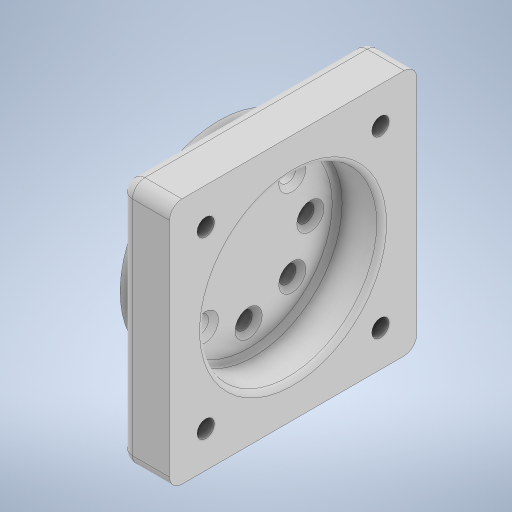
# Autodesk Inventor part: adaptador para Kuka
Saved by Autodesk Inventor 2024 (Build 280153000, 153)
## iProperties
Created: 2026-04-16
Part Number: adaptador para Kuka
Material: Genérico
Document SubType Name: Modeling
Designer: Legion
Density: 1 g/cm^3
Appearance: Valor por defecto
Author: Legion
Autodesk Inventor part; units mm, degrees
ref_plane "YZ Plane" through (0, 0, 0) normal (1, 0, 0) x (0, 1, 0)
ref_plane "XZ Plane" through (0, 0, 0) normal (0, 1, 0) x (-1, 0, 0)
ref_plane "XY Plane" through (0, 0, 0) normal (0, 0, 1) x (1, 0, 0)
sketch "Boceto1" plane through (0, 0, 0) normal (1, 0, 0) x (0, 1, 0)
  circle A0 centre (0, 0) radius 31.7
  circle A1 centre (0, 0) radius 40
  dimension "d0" = 63.4
  dimension "d1" = 80
  constraints: 2 centre point, 2 coincident
  measures "d0" diameter of A0
  measures "d1" diameter of A1
extrude "Extrusión1" add sketch "Boceto1" along normal blind 10 contours A0 | A1
extrude "Extrusión2" cut sketch "Boceto1" along normal blind 5 contours A0
sketch "Boceto2" plane through (10, 0, 0) normal (1, 0, 0) x (0, 0, -1)
  line L0 (0, 0) -> (50, 0)
  line L1 (0, 0) -> (-50, 0)
  line L2 (0, 0) -> (0, -50)
  line L3 (0, 0) -> (0, 50)
  line L4 (50, 50) -> (-50, 50)
  line L5 (-50, 50) -> (-50, -50)
  line L6 (-50, -50) -> (50, -50)
  line L7 (50, -50) -> (50, 50)
  dimension "d6" = 50
  dimension "d7" = 50
  dimension "d8" = 50
  dimension "d9" = 50
  constraints: 16 end point, 3 horizontal, 2 parallel, 2 perpendicular, 1 vertical
  measures "d6" distance of L0.start L0.end
  measures "d7" distance of L0.start L1.end
  measures "d8" distance of L0.start L2.end
  measures "d9" distance of L0.start L3.end
extrude "Extrusión3" add sketch "Boceto2" along normal blind 20
sketch "Boceto3" plane through (30, 0, 0) normal (1, 0, 0) x (0, 0, -1)
  circle A0 centre (0, 0) radius 31.7 projected
  circle A1 centre (0, 0) radius 40 projected
  circle A2 centre (0, 0) radius 31.7 projected
  line L0 (31.7, 0) -> (40, 0)
  circle A3 centre (0, 0) radius 35.85
  constraints: 2 end point, 2 horizontal alignment, 1 centre point, 1 coincident, 1 horizontal, 2 other
extrude "Extrusión4" cut sketch "Boceto3" against normal blind 18 contours A0 | A3
sketch "Boceto4" plane through (12, 0, 0) normal (1, 0, 0) x (0, 0, -1)
  circle A0 centre (0, 0) radius 25
  line L0 (-17.6777, -17.6777) -> (17.6777, 17.6777)
  line L1 (0, 0) -> (25, 0) construction
  line L2 (-17.6777, 17.6777) -> (17.6777, -17.6777)
  point P0 (0, -25)
  point P1 (-25, 0)
  point P2 (0, 25)
  dimension "d14" = 50
  dimension "d15" = 45
  constraints: 6 coincident, 6 end point, 2 midpoint, 1 horizontal, 9 other
  measures "d15" angle of L1 L0
hole "Agujero1" at (12, 17.6777, -17.6777) at (12, 0, -25) at (12, -17.6777, -17.6777) at (12, -25, 0) at (12, -17.6777, 17.6777) at (12, 0, 25) at (12, 17.6777, 17.6777) at (12, 25, 0) direction (-1, 0, 0) diameter 7 end through all countersink diameter 11 countersink angle 90
sketch "Boceto5" plane through (30, 0, 0) normal (1, 0, 0) x (0, 0, -1)
  circle A0 centre (0, 0) radius 50
  line L0 (50, 50) -> (-35.3553, -35.3553)
  line L1 (-35.3553, 35.3553) -> (50, -50)
  point P0 (35.3553, 35.3553)
  point P1 (-35.3553, -35.3553)
  point P2 (35.3553, -35.3553)
  constraints: 4 end point, 4 point on circle, 4 point on line, 3 coincident, 1 centre point
hole "Agujero2" at (30, 35.3553, -35.3553) at (30, 35.3553, 35.3553) at (30, -35.3553, 35.3553) at (30, -35.3553, -35.3553) direction (-1, 0, 0) diameter 7 end through all
sketch "Boceto6" plane through (10, 0, 0) normal (-1, 0, 0) x (0, 0, 1)
  circle A0 centre (-35.3553, -35.3553) radius 3.5
  line L0 (-37.6553, -39.3391) -> (-39.9553, -35.3553)
  line L1 (-39.9553, -35.3553) -> (-37.6553, -31.3716)
  line L2 (-37.6553, -31.3716) -> (-33.0553, -31.3716)
  line L3 (-33.0553, -31.3716) -> (-30.7553, -35.3553)
  line L4 (-30.7553, -35.3553) -> (-33.0553, -39.3391)
  line L5 (-33.0553, -39.3391) -> (-37.6553, -39.3391)
  line L6 (-35.3553, -35.3553) -> (-39.9553, -35.3553)
  circle A1 centre (-35.3553, 35.3553) radius 3.5
  circle A2 centre (35.3553, 35.3553) radius 3.5
  circle A3 centre (35.4038, -35.3068) radius 3.5
  line L7 (-37.6553, 31.3716) -> (-39.9553, 35.3553)
  line L8 (-33.0553, 31.3716) -> (-37.6553, 31.3716)
  line L9 (-30.7553, 35.3553) -> (-33.0553, 31.3716)
  line L10 (-33.0553, 39.3391) -> (-30.7553, 35.3553)
  line L11 (-37.6553, 39.3391) -> (-33.0553, 39.3391)
  line L12 (-39.9553, 35.3553) -> (-37.6553, 39.3391)
  line L13 (33.0553, 31.3716) -> (30.7553, 35.3553)
  line L14 (37.6553, 31.3716) -> (33.0553, 31.3716)
  line L15 (39.9553, 35.3553) -> (37.6553, 31.3716)
  line L16 (37.6553, 39.3391) -> (39.9553, 35.3553)
  line L17 (33.0553, 39.3391) -> (37.6553, 39.3391)
  line L18 (30.7553, 35.3553) -> (33.0553, 39.3391)
  line L19 (33.1038, -39.3391) -> (30.8038, -35.3553)
  line L20 (37.7038, -39.3391) -> (33.1038, -39.3391)
  line L21 (40.0038, -35.3553) -> (37.7038, -39.3391)
  line L22 (37.7038, -31.3716) -> (40.0038, -35.3553)
  line L23 (33.1038, -31.3716) -> (37.7038, -31.3716)
  line L24 (30.8038, -35.3553) -> (33.1038, -31.3716)
  line L25 (35.4038, -35.3553) -> (30.8038, -35.3553)
  circle A4 centre (35.3553, 35.3553) radius 3.5
  circle A5 centre (-35.3553, -35.3553) radius 3.5 projected
  point P0 (0, 0)
  point P1 (0, 0)
  point P2 (-50, -50)
  constraints: 52 end point, 12 parallel, 5 centre point
extrude "Extrusión5" cut sketch "Boceto6" against normal blind 6 contours L0 L1 L2 L3 L4 L5 | A1 | A2 | A3 | L7 L12 L11 L10 L9 L8 | L13 L18 L17 L16 L15 L14 | L19 L24 L23 L22 L21 L20
fillet "Empalme1" radius 1 2 edges at (5, -31.7, 0) (0, -31.7, 0)
fillet "Empalme2" radius 3 1 edges at (10, -40, 0)
fillet "Empalme3" radius 2 2 edges at (12, 0, 35.85) (30, 0, 35.85)
fillet "Empalme4" radius 5 8 edges at (20, -50, -50) (10, 0, -50) (10, -50, 0) (20, 50, -50) (10, 50, 0) (20, 50, 50) (10, 0, 50) (20, -50, 50)
